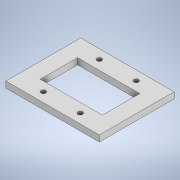
# Autodesk Inventor part: Viewing Mirror Holder Mount
Saved by Autodesk Inventor 2022 (Build 260153000, 153)
## iProperties
Created: 2023-09-18
Part Number: Viewing Mirror Holder Mount
Material: Generic
Document SubType Name: Modeling
Designer: fouad
Density: 1 g/cm^3
Appearance: Default
Author: fouad
Autodesk Inventor part; units mm, degrees
ref_plane "YZ Plane" through (0, 0, 0) normal (1, 0, 0) x (0, 1, 0)
ref_plane "XZ Plane" through (0, 0, 0) normal (0, 1, 0) x (-1, 0, 0)
ref_plane "XY Plane" through (0, 0, 0) normal (0, 0, 1) x (1, 0, 0)
sketch "Sketch1" plane through (0, 0, 0) normal (0, 1, 0) x (-1, 0, 0)
  line L0 (4.7412, 10.4222) -> (-10.2588, 10.4222)
  line L1 (-10.2588, 10.4222) -> (-10.2588, -1.5778)
  line L2 (-10.2588, -1.5778) -> (4.7412, -1.5778)
  line L3 (4.7412, -1.5778) -> (4.7412, 10.4222)
  line L4 (2.2412, 7.4222) -> (-7.7588, 7.4222)
  line L5 (-7.7588, 7.4222) -> (-7.7588, 1.4222)
  line L6 (-7.7588, 1.4222) -> (2.2412, 1.4222)
  line L7 (2.2412, 1.4222) -> (2.2412, 7.4222)
  circle A0 centre (0.2287, 8.9222) radius 0.375
  circle A1 centre (-5.6963, 8.9222) radius 0.375
  circle A2 centre (0.2287, -0.0628) radius 0.375
  circle A3 centre (-5.6963, -0.0628) radius 0.375
  point P0 (0, 0)
  dimension "d0" = 15
  dimension "d1" = 12
  dimension "d2" = 10
  dimension "d3" = 6
  dimension "d4" = 2.5
  dimension "d5" = 3
  dimension "d6" = 0.75
  dimension "d7" = 4.5125
  dimension "d8" = 1.5
  dimension "d11" = 5.925
  dimension "d14" = 8.985
  constraints: 16 end point, 4 centre point, 4 parallel, 3 horizontal, 2 perpendicular, 1 vertical, 6 other
  measures "d0" distance of L2.end L1.end
  measures "d1" distance of L1.end L0.end
  measures "d2" distance of L6.end L5.end
  measures "d3" distance of L5.end L4.end
  measures "d4" distance between parallel lines of L7 L3
  measures "d5" distance between parallel lines of L0 L4
  measures "d6" diameter of A0
  measures "d7" distance from line of L3 A0.centre
  measures "d8" distance from line of A0.centre L0
  measures "d11" distance of A0.centre A1.centre
  measures "d14" distance of A0.centre A2.centre
extrude "Extrusion1" add sketch "Sketch1" along normal blind 1
body "Solid1"
